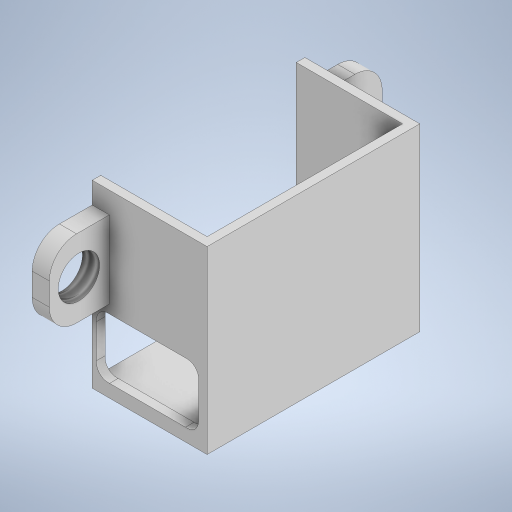
# Autodesk Inventor part: Servo Mount
Saved by Autodesk Inventor 2024.3 (Build 283343000, 343)
## iProperties
Created: 2026-02-23
Part Number: Servo Mount
Material: Generic
Document SubType Name: Modeling
Designer: nkt69613
Density: 1 g/cm^3
Appearance: Default
Author: nkt69613
Autodesk Inventor part; units mm, degrees
ref_plane "YZ Plane" through (0, 0, 0) normal (1, 0, 0) x (0, 1, 0)
ref_plane "XZ Plane" through (0, 0, 0) normal (0, 1, 0) x (-1, 0, 0)
ref_plane "XY Plane" through (0, 0, 0) normal (0, 0, 1) x (1, 0, 0)
sketch "Sketch1" plane through (0, 0, 0) normal (0, 1, 0) x (-1, 0, 0)
  line L0 (0, 0) -> (0, -22.8)
  line L1 (0, 0) -> (12.4, 0)
  line L2 (12.4, 0) -> (12.4, -22.8)
  line L3 (12.4, -22.8) -> (0, -22.8)
  line L4 (12.4, 0) -> (12.4, 1)
  line L5 (12.4, -22.8) -> (12.4, -23.8)
  line L6 (0, 0) -> (-1, 0)
  line L7 (12.4, 1) -> (-1, 1)
  line L8 (-1, 1) -> (-1, -23.8)
  line L9 (-1, -23.8) -> (12.4, -23.8)
  dimension "d0" = 22.8
  dimension "d1" = 12.4
  dimension "d2" = 1
  dimension "d3" = 1
  constraints: 20 end point, 3 horizontal, 3 perpendicular, 3 vertical, 1 parallel
  measures "d0" distance of L0.start L0.end
  measures "d1" distance of L0.start L1.end
  measures "d2" distance of L1.end L4.end
  measures "d3" distance of L2.end L5.end
extrude "Extrusion1" add sketch "Sketch1" along normal blind 21 contours L6 L8 L7 L4 L1 | L0 L3 L5 L9 L8 L6
sketch "Sketch2" plane through (-12.4, 0, -22.8) normal (0, 0, 1) x (1, 0, 0)
  line L0 (0, 0) -> (0, 21) projected
  line L1 (0, 0) -> (0, 1)
  line L2 (0, 1) -> (12.4, 1)
  line L3 (12.4, 0) -> (12.4, 21) projected
  line L4 (12.4, 0) -> (0, 0)
  dimension "d7" = 1
  constraints: 6 end point, 2 point on line, 1 horizontal, 1 parallel
  measures "d7" distance of L0.start L1.end
extrude "Extrusion2" add sketch "Sketch2" along normal blind 22.9
sketch "Sketch3" plane through (-12.4, 0, 1) normal (0, 0, 1) x (1, 0, 0)
  line L0 (12.4, 1) -> (0, 1) projected
  line L1 (0, 1) -> (0, 9)
  line L2 (0, 0) -> (0, 21) projected
  line L3 (0, 9) -> (13.4, 9)
  line L4 (13.4, 0) -> (13.4, 21) projected
  line L5 (13.4, 1) -> (13.4, 9)
  line L6 (13.4, 1) -> (0, 1)
  line L7 (0.5, 8.5) -> (0.5, 1.5)
  line L8 (0, 0) -> (13.4, 0) projected
  line L9 (0.5, 8.5) -> (12.9, 8.5)
  line L10 (12.4, 1) -> (12.4, 21) projected
  line L11 (12.9, 8.5) -> (12.9, 1.5)
  line L12 (12.9, 1.5) -> (0.5, 1.5)
  point P0 (12.4, 0)
  point P1 (12.4, 1.5)
  point P2 (12.4, 8.5)
  dimension "d10" = 8
  constraints: 16 end point, 6 perpendicular, 3 point on line, 1 collinear
  measures "d10" distance of L0.end L1.end
extrude "Extrusion3" cut sketch "Sketch3" against normal blind 1 contours L12 L7 L9 L10
sketch "Sketch4" plane through (-12.4, 0, 1) normal (0, 0, 1) x (1, 0, 0)
  line L0 (12.4, 8.5) -> (0.5, 8.5) projected
  line L1 (2, 9.5) -> (2, 18.5)
  line L2 (2, 18.5) -> (0, 18.5)
  line L3 (0, 1) -> (0, 21) projected
  line L4 (2, 9.5) -> (0, 9.5)
  point P0 (12.4, 0)
  dimension "d20" = 9
  constraints: 6 end point, 2 point on line, 1 horizontal, 1 perpendicular, 1 vertical
  measures "d20" distance of L1.start L1.end
extrude "Extrusion4" add sketch "Sketch4" along normal blind 7
sketch "Sketch5" plane through (1, 0, -23.8) normal (0, 0, -1) x (-1, 0, 0)
  line L0 (0, 0) -> (13.4, 0) projected
  line L1 (13.4, 0) -> (13.4, 9.398)
  line L2 (13.4, 0) -> (13.4, 21) projected
  line L3 (13.4, 9.398) -> (13.4, 18.3896)
  line L4 (13.4, 18.3896) -> (11.3934, 18.3896)
  line L5 (11.3934, 18.3896) -> (11.3934, 9.398)
  line L6 (11.3934, 9.398) -> (13.4, 9.398)
  point P0 (1, 0)
  dimension "d24" = 9.398
  dimension "d25" = 8.9916
  dimension "d26" = 2.0066
  constraints: 10 end point, 3 perpendicular, 2 point on line
  measures "d24" distance of L0.end L1.end
  measures "d25" distance of L1.end L3.end
  measures "d26" distance of L3.end L4.end
extrude "Extrusion5" add sketch "Sketch5" along normal blind 7
fillet "Fillet1" radius 3.175 4 edges at (-11.4, 18.5, 8) (-11.4, 9.5, 8) (-11.3967, 18.3896, -30.8) (-11.3967, 9.398, -30.8)
sketch "Sketch6" plane through (-10.4, 9.5, 1) normal (1, 0, 0) x (0, 0, -1)
  line L0 (0, 9) -> (-3.556, 9)
  line L1 (0, 9) -> (-3.825, 9) projected
  line L2 (-3.556, 9) -> (-3.556, 4.5042)
  line L3 (24.8, 8.8896) -> (28.625, 8.8896) projected
  circle A0 centre (-3.556, 4.5042) radius 2.413
  point P0 (1, -9.5)
  dimension "d33" = 3.556
  dimension "d34" = 4.4958
  dimension "d37" = 4.826
  constraints: 4 end point, 1 centre point, 1 coincident, 1 perpendicular, 1 point on line
  measures "d33" distance of L0.start L0.end
  measures "d34" distance of L0.end L2.end
  measures "d37" diameter of A0
extrude "Extrusion6" cut sketch "Sketch6" against normal blind 7
thread "Thread1" size "10-24 UNC" class "2B" standard "ANSI Unified Screw Threads" full length
sketch "Sketch7" plane through (-10.3934, 9.398, -23.8) normal (1, 0, 0) x (0, 0, -1)
  line L0 (0, 8.9916) -> (3.556, 8.9916)
  line L1 (0, 8.9916) -> (3.825, 8.9916) projected
  line L2 (3.556, 8.9916) -> (3.556, 4.4958)
  circle A0 centre (3.556, 4.4958) radius 2.413
  point P0 (-23.8, -9.398)
  dimension "d42" = 3.556
  dimension "d43" = 4.4958
  dimension "d44" = 4.826
  constraints: 4 end point, 1 centre point, 1 coincident, 1 perpendicular, 1 point on line
  measures "d42" distance of L0.start L0.end
  measures "d43" distance of L0.end L2.end
  measures "d44" diameter of A0
extrude "Extrusion7" cut sketch "Sketch7" against normal blind 7
thread "Thread2" size "10-24 UNC" class "2B" standard "ANSI Unified Screw Threads" full length
fillet "Fillet2" radius 1.524 4 edges at (-11.9, 8.5, 0.5) (0, 8.5, 0.5) (0, 1.5, 0.5) (-11.9, 1.5, 0.5)
body "Solid1"
